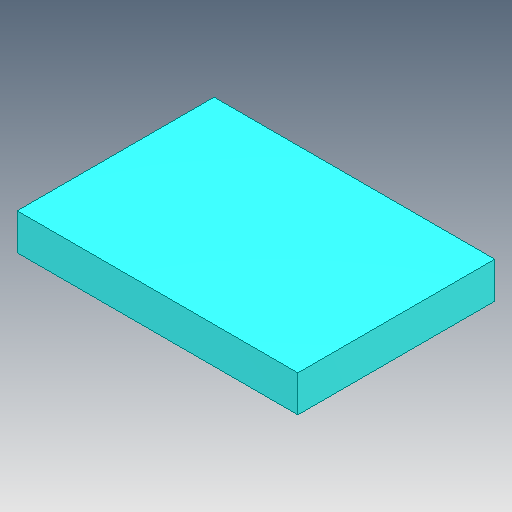
# Autodesk Inventor part: ISP
Saved by Autodesk Inventor 2017 (Build 210142000, 142)
## iProperties
Part Number: ISP
Material: Generisch
Document SubType Name: Modeling
Designer: Werkstatt
Density: 1 g/cm^3
Appearance: 2X3, ISP
Author: Werkstatt
Autodesk Inventor part; units mm, degrees
ref_plane "YZ Plane" through (0, 0, 0) normal (1, 0, 0) x (0, 1, 0)
ref_plane "XZ Plane" through (0, 0, 0) normal (0, 1, 0) x (-1, 0, 0)
ref_plane "XY Plane" through (0, 0, 0) normal (0, 0, 1) x (1, 0, 0)
sketch "2X3, ISP_27" plane through (0, 0, 0) normal (0, 0, 1) x (1, 0, 0)
  line L0 (-1.3716, 3.81) -> (6.35, 3.81)
  line L1 (6.35, 3.81) -> (6.35, -1.605)
  line L2 (6.35, -1.605) -> (-1.3716, -1.605)
  line L3 (-1.3716, -1.605) -> (-1.3716, 3.81)
  constraints: 8 end point
extrude "Extrusion1" add sketch "2X3, ISP_27" along normal blind 1
